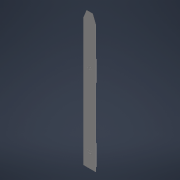
# Autodesk Inventor part: PlanchaHorqSup
Saved by Autodesk Inventor 2022 (Build 260153000, 153)
## iProperties
Created: 2021-09-29
Part Number: PlanchaHorqSup
Material: Steel, Galvanized
Document SubType Name: Sheet Metal
Designer: Andres
Mass: 9380.75 g
Surface Area: 4929.77 cm^2
Volume: 1195 cm^3
Density: 7.85 g/cm^3
Sheet Metal Rule: thin_mm
Appearance: Galvanized
Author: Andres
Autodesk Inventor part; units mm, degrees
ref_plane "YZ Plane" through (0, 0, 0) normal (1, 0, 0) x (0, 1, 0)
ref_plane "XZ Plane" through (0, 0, 0) normal (0, 1, 0) x (-1, 0, 0)
ref_plane "XY Plane" through (0, 0, 0) normal (0, 0, 1) x (1, 0, 0)
sketch "Sketch3" plane through (0, 0, 8) normal (0, 0, 1) x (1, 0, 0)
  line L0 (45, 240) -> (165, 240)
  line L1 (165, 750) -> (45, 750)
  line L2 (45, 0) -> (45, 1244.2225)
  line L3 (165, 1244.2225) -> (165, 0)
  line L4 (45, 950) -> (165, 950)
  line L5 (45, 0) -> (45, 1244.2225)
  line L6 (45, 1244.2225) -> (75.311, 1320)
  line L7 (75.311, 1320) -> (134.689, 1320)
  line L8 (134.689, 1320) -> (165, 1244.2225)
  line L9 (165, 1244.2225) -> (165, 0)
  line L10 (165, 40) -> (45, 40)
  line L11 (45, 0) -> (45, 1244.2225)
  line L12 (165, 1244.2225) -> (165, 0)
  line L13 (15, 0) -> (195, 0) construction
  line L14 (45, 0) -> (165, 0)
  point P0 (0, 0)
sketch "Sketch1" plane through (0, 0, 0) normal (0, 0, 1) x (1, 0, 0)
  line L0 (15, 1250) -> (15, 0) construction
  line L1 (195, 1250) -> (195, 0) construction
  line L2 (15, 0) -> (195, 0) construction
  line L3 (15, 1250) -> (55, 1350) construction
  line L4 (55, 1350) -> (155, 1350) construction
  line L5 (155, 1350) -> (195, 1250) construction
  line L6 (15, 360) -> (195, 360)
  line L7 (15, 630) -> (195, 630)
  line L8 (15, 140) -> (195, 140) construction
  line L9 (15, 850) -> (195, 850) construction
  line L10 (165, 750) -> (45, 750)
  line L11 (45, 750) -> (45, 950)
  line L12 (45, 950) -> (165, 950)
  line L13 (165, 950) -> (165, 750)
  line L14 (165, 750) -> (45, 950) construction
  line L15 (45, 750) -> (165, 950) construction
  line L16 (45, 0) -> (45, 1244.2225)
  line L17 (45, 1244.2225) -> (75.311, 1320)
  line L18 (75.311, 1320) -> (134.689, 1320)
  line L19 (134.689, 1320) -> (165, 1244.2225)
  line L20 (165, 1244.2225) -> (165, 0)
  line L21 (45, 40) -> (165, 40)
  line L22 (165, 40) -> (165, 240)
  line L23 (165, 240) -> (45, 240)
  line L24 (45, 240) -> (45, 40)
  line L25 (45, 40) -> (165, 240) construction
  line L26 (165, 40) -> (45, 240) construction
  line L27 (105, 0) -> (105, 1320) construction
  point P0 (105, 850)
  point P1 (105, 140)
  dimension "d11" = 30
  dimension "d12" = 200
  dimension "d13" = 200
  measures "d11" distance between parallel lines of L0 L16
  measures "d12" distance between parallel lines of L12 L10
  measures "d13" distance between parallel lines of L23 L21
extrude "Plate1" add sketch "Sketch1" along normal blind 8 contours L23 L20 L21 L16 | L11 L12 L13 L10
sketch "Sketch2" plane through (0, 0, 8) normal (0, 0, 1) x (1, 0, 0)
  circle A0 centre (118.8564, 132.3929) radius 1.621 projected
  circle A1 centre (105, 124.3929) radius 1.621 projected
  circle A2 centre (118.8564, 148.3929) radius 1.621 projected
  circle A3 centre (118.8564, 132.3929) radius 1.621 projected
  circle A4 centre (105, 124.3929) radius 1.621 projected
  circle A5 centre (91.1436, 132.3929) radius 1.621 projected
  circle A6 centre (91.1436, 148.3929) radius 1.621 projected
  circle A7 centre (105, 156.3929) radius 1.621 projected
  circle A8 centre (118.8564, 841.6071) radius 1.621 projected
  circle A9 centre (105, 833.6071) radius 1.621 projected
  circle A10 centre (91.1436, 841.6071) radius 1.621 projected
  line L0 (165, 630) -> (165, 960) projected
  line L1 (45, 630) -> (165, 630) projected
  line L2 (45, 960) -> (45, 630) projected
  line L3 (165, 960) -> (45, 960) projected
  circle A11 centre (91.1436, 857.6071) radius 1.621 projected
  circle A12 centre (91.1436, 841.6071) radius 1.621 projected
  circle A13 centre (118.8564, 841.6071) radius 1.621 projected
  circle A14 centre (105, 833.6071) radius 1.621 projected
  circle A15 centre (91.1436, 857.6071) radius 1.621 projected
  circle A16 centre (105, 865.6071) radius 1.621 projected
  circle A17 centre (118.8564, 857.6071) radius 1.621 projected
  point P0 (0, 0)
hole "Hole1" at (118.8564, 132.3929, 8) at (105, 124.3929, 8) at (91.1436, 132.3929, 8) at (91.1436, 148.3929, 8) at (105, 156.3929, 8) at (118.8564, 148.3929, 8) at (105, 833.6071, 8) at (91.1436, 841.6071, 8) at (91.1436, 857.6071, 8) at (118.8564, 841.6071, 8) at (118.8564, 857.6071, 8) at (105, 865.6071, 8) direction (0, 0, -1) diameter 4.5 end through all counterbore diameter 8 counterbore depth 4.6 clearance for "Socket Head Cap Screw ISO 4762" size "M4" standard "ISO"
extrude "Plate2" add sketch "Sketch3" against normal blind 2 separate body contours L2 L1 L3 L0 | L10 L3 L14 L2 | L2 L6 L7 L8 L3 L4
equation "\"d13\" = d12"
equation "\"d9\" = Thickness"
equation "\"d14\" = Thickness"
equation "\"BendRadius\" = Thickness"
equation "\"BendReliefWidth\" = Thickness"
equation "\"BendReliefDepth\" = 0.5 * Thickness"
equation "\"CornerReliefSize\" = 4 * Thickness"
equation "\"MinimumRemnant\" = 2 * Thickness"
equation "\"TransitionRadius\" = BendRadius"
equation "\"JacobiRadiusSize\" = BendRadius"
equation "\"GapSize\" = Thickness"
body "Solid1"
body "Solid2"
